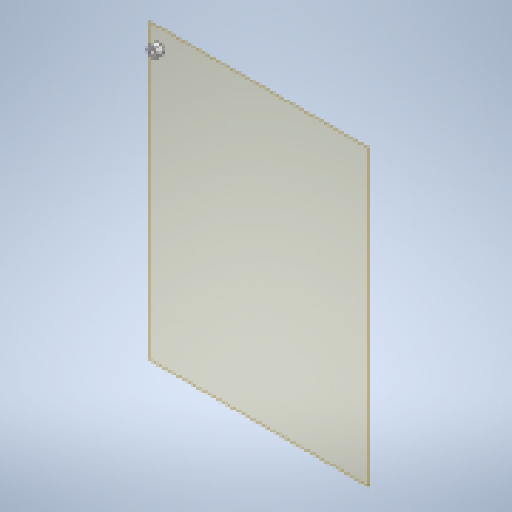
# Autodesk Inventor part: spacing-nuts
Saved by Autodesk Inventor 2023 (Build 270158030, 158C)
## iProperties
Created: 2024-04-01
Part Number: spacing-nuts
Material: Generic
Document SubType Name: Modeling
Designer: Imogen Heard
Density: 1 g/cm^3
Appearance: Default
Author: Imogen Heard
Autodesk Inventor part; units mm, degrees
ref_plane "YZ Plane" through (0, 0, 0) normal (1, 0, 0) x (0, 1, 0)
ref_plane "XZ Plane" through (0, 0, 0) normal (0, 1, 0) x (-1, 0, 0)
ref_plane "Work Plane1" through (205.1053, 785.1546, 0) normal (0, 0, 1) x (1, 0, 0)
sketch "Sketch1" plane through (205.1053, 785.1546, 0) normal (0, 0, 1) x (1, 0, 0)
  line L0 (-184.8449, 223.82) -> (-179.9374, 232.32)
  line L1 (-179.9374, 232.32) -> (-170.1225, 232.32)
  line L2 (-170.1225, 232.32) -> (-165.215, 223.82)
  line L3 (-165.215, 223.82) -> (-170.1225, 215.32)
  line L4 (-170.1225, 215.32) -> (-179.9374, 215.32)
  line L5 (-179.9374, 215.32) -> (-184.8449, 223.82)
  circle A0 centre (-175.0299, 223.82) radius 3.7
  point P0 (-205.1053, -785.1546)
  dimension "d0" = 17
  dimension "d1" = 7.4
  constraints: 12 end point, 1 centre point, 1 coincident, 1 horizontal, 13 other
  measures "d0" distance between parallel lines of L2 L5
  measures "d1" diameter of A0
extrude "Extrusion1" add sketch "Sketch1" along normal blind 11.85
body "Solid1"
